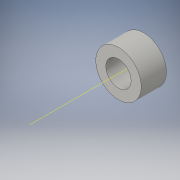
# Autodesk Inventor part: Caufield_Hitch_Magnet
Saved by Autodesk Inventor 2016 (Build 200138000, 138)
## iProperties
Created: 2018-01-08
Part Number: Caufield_Hitch_Magnet
Material: Generic
Document SubType Name: Modeling
Designer: caufield58738
Density: 1 g/cm^3
Appearance: Default
Author: caufield58738
Autodesk Inventor part; units mm, degrees
ref_plane "YZ Plane" through (0, 0, 0) normal (1, 0, 0) x (0, 1, 0)
ref_plane "XZ Plane" through (0, 0, 0) normal (0, 1, 0) x (-1, 0, 0)
ref_plane "XY Plane" through (0, 0, 0) normal (0, 0, 1) x (1, 0, 0)
sketch "Hitch Magnet Sketch" plane through (0, 0, 0) normal (0, 0, 1) x (1, 0, 0)
  circle A0 centre (0, 0) radius 5.715
  dimension "d0" = 11.43
  constraints: 2 coincident, 1 centre point
  measures "d0" diameter of A0
extrude "Hitch Magnet Extrution" add sketch "Hitch Magnet Sketch" along normal blind 6.35
hole "Hitch Magnet Hole" at (0, 0, 0) direction (0, 0, 1) diameter 6.35 end through all
body "Solid1"
